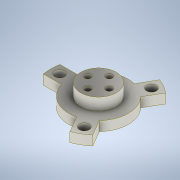
# Autodesk Inventor part: Planet_Gear_Output
Saved by Autodesk Inventor 2022 (Build 260153000, 153)
## iProperties
Created: 2022-04-22
Part Number: Planet_Gear_Output
Material: Generic
Document SubType Name: Modeling
Designer: Mlees
Density: 1 g/cm^3
Appearance: Silver
Mass: 4.19966 g
Surface Area: 23.4388 cm^2
Volume: 4.19966 cm^3
Author: Mlees
Autodesk Inventor part; units mm, degrees
ref_plane "YZ Plane" through (0, 0, 0) normal (1, 0, 0) x (0, 1, 0)
ref_plane "XZ Plane" through (0, 0, 0) normal (0, 1, 0) x (-1, 0, 0)
ref_plane "XY Plane" through (0, 0, 0) normal (0, 0, 1) x (1, 0, 0)
sketch "Sketch1" plane through (0, 0, 0) normal (0, 1, 0) x (-1, 0, 0)
  circle A0 centre (16.272, 0) radius 2.1
  line L0 (14.741, 3.5) -> (19.6914, 3.5)
  line L1 (14.741, -3.5) -> (19.6914, -3.5)
  line L2 (14.741, 3.5) -> (12, 3.5)
  line L3 (14.741, -3.5) -> (12, -3.5)
  line L4 (-2.9689, 12.1423) -> (-6.8146, 18.8032)
  line L5 (-12.8768, 15.3032) -> (-9.0311, 8.6423)
  line L6 (12, -3.5) -> (19.6914, -3.5)
  line L7 (12, 3.5) -> (19.6914, 3.5)
  line L8 (-2.9689, -12.1423) -> (-6.8146, -18.8032)
  line L9 (-9.0311, -8.6423) -> (-12.8768, -15.3032)
  arc A1 (-6.8146, 18.8032) -> (-12.8768, 15.3032) centre (0, 0) ccw
  arc A2 (-12.8768, -15.3032) -> (-6.8146, -18.8032) centre (0, 0) ccw
  arc A3 (19.6914, -3.5) -> (19.6914, 3.5) centre (0, 0) ccw
  arc A4 (-9.0311, 8.6423) -> (-9.0311, -8.6423) centre (0, 0) ccw
  arc A5 (-2.9689, -12.1423) -> (12, -3.5) centre (0, 0) ccw
  arc A6 (12, 3.5) -> (-2.9689, 12.1423) centre (0, 0) ccw
  line L10 (0, 0) -> (16.272, 0)
  circle A7 centre (-8.136, 14.092) radius 2.1
  circle A8 centre (-8.136, -14.092) radius 2.1
  dimension "d6" = 4.2
  dimension "d20" = 16.272
  dimension "d23" = 360
  constraints: 22 end point, 12 point on circle, 9 centre point, 3 horizontal, 1 coincident, 1 collinear, 1 parallel, 7 other
  measures "d6" diameter of A0
  measures "d20" distance of L10.start L10.end
extrude "Extrusion1" add sketch "Sketch1" along normal blind 4
sketch "Sketch2" plane through (0, 4, 0) normal (0, 1, 0) x (1, 0, 0)
  circle A0 centre (0, 0) radius 7.5
  constraints: 1 centre point, 1 coincident
extrude "Extrusion2" add sketch "Sketch2" along normal blind 5
sketch "Sketch3" plane through (0, 9, 0) normal (0, 1, 0) x (1, 0, 0)
  circle A0 centre (-4.5, 0) radius 1.35
  circle A1 centre (0, -4.5) radius 1.35
  circle A2 centre (4.5, 0) radius 1.35
  circle A3 centre (0, 4.5) radius 1.35
  point P0 (0, 0)
  point P1 (0, 0)
  dimension "d26" = 2.7
  dimension "d30" = 360
  constraints: 4 centre point, 1 coincident, 9 other
  measures "d26" diameter of A0
extrude "Extrusion3" cut sketch "Sketch3" against normal through all
sketch "Sketch4" plane through (0, 0, 0) normal (0, -1, 0) x (1, 0, 0)
  circle A0 centre (-4.5, 0) radius 1.35 projected
  circle A1 centre (-4.5, 0) radius 2
  circle A2 centre (0, -4.5) radius 2
  circle A3 centre (4.5, 0) radius 2
  circle A4 centre (0, 4.5) radius 2
  point P0 (0, 0)
  point P1 (0, 0)
  dimension "d34" = 4
  dimension "d37" = 360
  constraints: 4 centre point, 2 coincident, 9 other
  measures "d34" diameter of A1
extrude "Extrusion4" cut sketch "Sketch4" against normal blind 3
body "Solid1"
